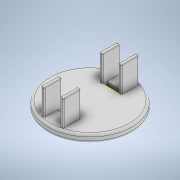
# Autodesk Inventor part: TAPPO
Saved by Autodesk Inventor 2022 (Build 260153000, 153)
## iProperties
Created: 2022-03-20
Part Number: TAPPO
Material: Generico
Document SubType Name: Modeling
Designer: dutto
Density: 1 g/cm^3
Appearance: Default
Author: dutto
Autodesk Inventor part; units mm, degrees
ref_plane "YZ Plane" through (0, 0, 0) normal (1, 0, 0) x (0, 1, 0)
ref_plane "XZ Plane" through (0, 0, 0) normal (0, 1, 0) x (-1, 0, 0)
ref_plane "XY Plane" through (0, 0, 0) normal (0, 0, 1) x (1, 0, 0)
sketch "Schizzo1" plane through (0, 0, 0) normal (0, 1, 0) x (-1, 0, 0)
  circle A0 centre (0, 0) radius 37
  dimension "d0" = 74
  constraints: 1 centre point, 1 coincident
  measures "d0" diameter of A0
extrude "Estrusione1" add sketch "Schizzo1" along normal blind 7
fillet "Raccordo1" radius 2 1 edges at (37, 7, 0)
fillet "Raccordo2" radius 2 1 edges at (37, 0, 0)
sketch "Schizzo2" plane through (0, 7, 0) normal (0, 1, 0) x (1, 0, 0)
  circle A0 centre (0, 0) radius 35 projected
  line L0 (0, -18.5) -> (-6.35, -18.5)
  line L1 (0, -18.5) -> (6.35, -18.5)
  line L2 (-6.35, -18.5) -> (-6.35, -21.5)
  line L3 (-6.35, -21.5) -> (6.35, -21.5)
  line L4 (6.35, -21.5) -> (6.35, -18.5)
  line L5 (0, 18.5) -> (-6.35, 18.5)
  line L6 (0, 18.5) -> (6.35, 18.5)
  line L7 (-6.35, 18.5) -> (-6.35, 21.5)
  line L8 (-6.35, 21.5) -> (6.35, 21.5)
  line L9 (6.35, 21.5) -> (6.35, 18.5)
  dimension "d10" = 6.35
  dimension "d12" = 3
  constraints: 20 end point, 2 perpendicular, 2 point on line, 1 horizontal, 1 vertical
  measures "d10" distance of L0.start L0.end
  measures "d12" distance of L0.end L2.end
extrude "Estrusione2" cut sketch "Schizzo2" against normal blind 3 contours L1 L4 L3 L2 L0 | L5 L7 L8 L9 L6
fillet "Raccordo3" radius 0.5 8 edges at (0, 7, 18.5) (0, 7, 21.5) (-6.35, 7, 20) (6.35, 7, 20) (0, 7, -18.5) (-6.35, 7, -20) (0, 7, -21.5) (6.35, 7, -20)
sketch "Schizzo3" plane through (0, 7, 0) normal (0, 1, 0) x (1, 0, 0)
  line L0 (-6.85, -18) -> (-6.85, -22) projected
  line L1 (-6.85, -18) -> (-9.85, -18)
  line L2 (-9.85, -18) -> (-9.85, -33.5)
  line L3 (-9.85, -33.5) -> (-6.85, -33.5)
  line L4 (-6.85, -33.5) -> (-6.85, -18)
  line L5 (6.85, -18) -> (-6.85, -18) projected
  line L6 (6.85, -18) -> (9.85, -18)
  line L7 (9.85, -18) -> (9.85, -33.5)
  line L8 (9.85, -33.5) -> (6.85, -33.5)
  line L9 (6.85, -33.5) -> (6.85, -18)
  line L10 (-6.85, 18) -> (-9.85, 18)
  line L11 (-9.85, 18) -> (-9.85, 33.5)
  line L12 (-9.85, 33.5) -> (-6.85, 33.5)
  line L13 (-6.85, 33.5) -> (-6.85, 18)
  line L14 (9.85, 18) -> (9.85, 33.5)
  line L15 (9.85, 33.5) -> (6.85, 33.5)
  line L16 (6.85, 33.5) -> (6.85, 18)
  line L17 (6.85, 18) -> (9.85, 18)
  point P0 (0, 0)
  dimension "d16" = 15.5
  dimension "d17" = 3
  constraints: 32 end point, 2 parallel, 1 horizontal, 1 perpendicular
  measures "d16" distance of L1.end L2.end
  measures "d17" distance of L0.start L1.end
extrude "Estrusione3" add sketch "Schizzo3" along normal blind 22.5
fillet "Raccordo4" radius 1 16 edges at (9.85, 18.25, 18) (-6.85, 18.25, 18) (-9.85, 18.25, 18) (6.85, 18.25, 18) (9.85, 18.25, -18) (6.85, 18.25, -18) (-6.85, 18.25, -18) (-9.85, 18.25, -18) (9.85, 18.25, -33.5) (6.85, 18.25, -33.5) (-6.85, 18.25, -33.5) (-9.85, 18.25, -33.5) (-9.85, 18.25, 33.5) (-6.85, 18.25, 33.5) (6.85, 18.25, 33.5) (9.85, 18.25, 33.5)
fillet "Raccordo5" radius 0.5 32 edges at (-9.5571, 29.5, 33.2071) (-8.35, 29.5, 33.5) (-7.1429, 29.5, 33.2071) (-6.85, 29.5, 25.75) (-7.1429, 29.5, 18.2929) (-8.35, 29.5, 18) (-9.5571, 29.5, 18.2929) (-9.85, 29.5, 25.75) (7.1429, 29.5, 33.2071) (8.35, 29.5, 33.5) (9.5571, 29.5, 33.2071) (9.85, 29.5, 25.75) (9.5571, 29.5, 18.2929) (8.35, 29.5, 18) (7.1429, 29.5, 18.2929) (6.85, 29.5, 25.75) (-9.5571, 29.5, -18.2929) (-8.35, 29.5, -18) (-7.1429, 29.5, -18.2929) (-6.85, 29.5, -25.75) (-7.1429, 29.5, -33.2071) (-8.35, 29.5, -33.5) (-9.5571, 29.5, -33.2071) (-9.85, 29.5, -25.75) (7.1429, 29.5, -18.2929) (8.35, 29.5, -18) (9.5571, 29.5, -18.2929) (9.85, 29.5, -25.75) (9.5571, 29.5, -33.2071) (8.35, 29.5, -33.5) (7.1429, 29.5, -33.2071) (6.85, 29.5, -25.75)
sketch "Schizzo4" plane through (0, 7, 0) normal (0, 1, 0) x (1, 0, 0)
  line L0 (-6.85, 18) -> (6.85, 18) projected
  line L1 (6.85, -18) -> (-6.85, -18) projected
